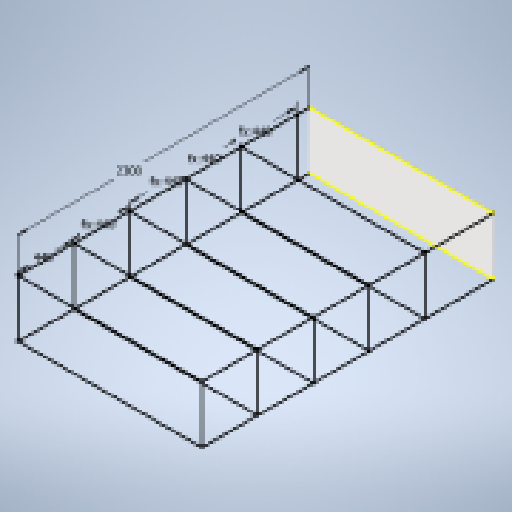
# Autodesk Inventor part: sketch-rack2
Saved by Autodesk Inventor 2023.2 (Build 272271030, 271C)
## iProperties
Created: 2023-08-24
Part Number: sketch-rack2
Material: Generic
Document SubType Name: Modeling
Designer: admin
Density: 1 g/cm^3
Appearance: Default
Author: admin
Autodesk Inventor part; units mm, degrees
ref_plane "YZ Plane" through (0, 0, 0) normal (1, 0, 0) x (0, 1, 0)
ref_plane "XZ Plane" through (0, 0, 0) normal (0, 1, 0) x (-1, 0, 0)
ref_plane "XY Plane" through (0, 0, 0) normal (0, 0, 1) x (1, 0, 0)
sketch "Sketch1" plane through (0, 0, 0) normal (0, 0, 1) x (1, 0, 0)
  line L0 (-725, 245) -> (725, 245)
  line L1 (725, 245) -> (725, -245)
  line L2 (725, -245) -> (-725, -245)
  line L3 (-725, -245) -> (-725, 245)
  line L4 (-725, 245) -> (725, -245) construction
  line L5 (725, 245) -> (-725, -245) construction
  line L6 (725, 225) -> (-725, 225)
  line L7 (-725, -225) -> (725, -225)
  point P0 (0, 0)
  dimension "d0" = 1450
  dimension "d1" = 490
  dimension "d2" = 20
  dimension "d6" = 20
  constraints: 16 end point, 4 point on line, 3 parallel, 2 midpoint, 1 horizontal, 1 perpendicular
  measures "d0" distance of L1.end L2.end
  measures "d1" distance of L0.end L1.end
  measures "d2" distance between parallel lines of L0 L6
  measures "d6" distance between parallel lines of L2 L7
extrude "Extrusion1" add sketch "Sketch1" against normal blind 10 contours L6 L1 L7 L3
sketch3d "3D Sketch1"
equation "\"d6\" = d2"
equation "\"d8\" = d7"
equation "\"d9\" = d7"
equation "\"d10\" = d7"
equation "\"d11\" = d7"
equation "\"d7\" = 440"
body "Solid1"
